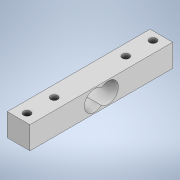
# Autodesk Inventor part: Mockup Load Cell (based on 1kg Adafruit)
Saved by Autodesk Inventor 2020 (Build 240168000, 168)
## iProperties
Created: 2022-03-09
Part Number: Mockup Load Cell (based on 1kg Adafruit)
Material: Generic
Document SubType Name: Modeling
Designer: kamer
Density: 1 g/cm^3
Appearance: Default
Author: kamer
Autodesk Inventor part; units mm, degrees
ref_plane "YZ Plane" through (0, 0, 0) normal (1, 0, 0) x (0, 1, 0)
ref_plane "XZ Plane" through (0, 0, 0) normal (0, 1, 0) x (-1, 0, 0)
ref_plane "XY Plane" through (0, 0, 0) normal (0, 0, 1) x (1, 0, 0)
sketch "Sketch1" plane through (0, 0, 0) normal (0, 0, 1) x (1, 0, 0)
  line L0 (0, 0) -> (12.7, 0)
  line L1 (12.7, 0) -> (12.7, 12.7)
  line L2 (12.7, 12.7) -> (0, 12.7)
  line L3 (0, 12.7) -> (0, 0)
  dimension "d0" = 12.7
  dimension "d1" = 12.7
  constraints: 8 end point, 2 parallel, 1 horizontal, 1 perpendicular
  measures "d0" distance of L2.end L1.end
  measures "d1" distance of L1.end L0.end
extrude "Extrusion1" add sketch "Sketch1" along normal blind 80.01
sketch "Sketch2" plane through (12.7, 0, 0) normal (1, 0, 0) x (0, 0, -1)
  circle A0 centre (-43.815, 6.35) radius 5.715
  circle A1 centre (-36.195, 6.35) radius 5.715
  line L0 (-43.815, 6.35) -> (-36.195, 6.35) construction
  line L1 (0, 12.7) -> (-80.01, 12.7) construction
  line L2 (-36.195, 6.35) -> (-40.005, 6.35) construction
  line L3 (-80.01, 0) -> (-80.01, 12.7) construction
  point P0 (0, 0)
  point P1 (-40.005, 10.6097)
  point P2 (-40.005, 2.0903)
  dimension "d4" = 11.43
  dimension "d5" = 11.43
  dimension "d6" = 6.35
  dimension "d7" = 7.62
  dimension "d8" = 40.005
  constraints: 4 end point, 2 centre point, 1 horizontal, 1 midpoint
  measures "d4" diameter of A0
  measures "d5" diameter of A1
  measures "d6" distance between parallel lines of L1 L0
  measures "d7" distance of L0.end L0.start
  measures "d8" distance from line of L3 L2.end
extrude "Extrusion2" cut sketch "Sketch2" against normal through all
sketch "Sketch3" plane through (0, 12.7, 0) normal (0, 1, 0) x (1, 0, 0)
  circle A0 centre (6.35, -75.311) radius 2
  line L0 (12.7, -80.01) -> (0, -80.01) projected
  line L1 (0, 0) -> (0, -80.01) projected
  circle A1 centre (6.35, -60.071) radius 2
  circle A2 centre (6.35, -4.699) radius 2
  circle A3 centre (6.35, -19.939) radius 2
  line L2 (12.7, 0) -> (0, 0) projected
  dimension "d11" = 4
  dimension "d12" = 4.699
  dimension "d13" = 6.35
  dimension "d14" = 4
  dimension "d15" = 15.24
  dimension "d16" = 6.35
  dimension "d17" = 4
  dimension "d18" = 4
  dimension "d19" = 6.35
  dimension "d20" = 6.35
  dimension "d21" = 4.699
  dimension "d22" = 15.24
  constraints: 4 centre point
  measures "d11" diameter of A0
  measures "d12" distance from line of L0 A0.centre
  measures "d13" distance from line of L1 A0.centre
  measures "d14" diameter of A1
  measures "d15" distance of A1.centre A0.centre
  measures "d16" distance from line of L1 A1.centre
  measures "d17" diameter of A2
  measures "d18" diameter of A3
  measures "d19" distance from line of L1 A2.centre
  measures "d20" distance from line of L1 A3.centre
  measures "d21" distance from line of L2 A2.centre
  measures "d22" distance of A2.centre A3.centre
extrude "Extrusion3" cut sketch "Sketch3" against normal through all
body "Solid1"
